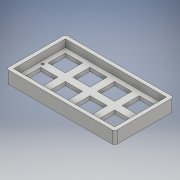
# Autodesk Inventor part: Key Plate
Saved by Autodesk Inventor 2018 (Build 220112000, 112)
## iProperties
Created: 2018-05-10
Part Number: Key Plate
Material: Generic
Document SubType Name: Modeling
Designer: mtsti
Density: 1 g/cm^3
Appearance: Default
Author: mtsti
Autodesk Inventor part; units mm, degrees
ref_plane "YZ Plane" through (0, 0, 0) normal (1, 0, 0) x (0, 1, 0)
ref_plane "XZ Plane" through (0, 0, 0) normal (0, 1, 0) x (-1, 0, 0)
ref_plane "XY Plane" through (0, 0, 0) normal (0, 0, 1) x (1, 0, 0)
sketch "Sketch1" plane through (0, 0, 0) normal (0, 0, 1) x (1, 0, 0)
  line L0 (3.0232, 17.5372) -> (17.0232, 17.5372)
  line L1 (17.0232, 17.5372) -> (17.0232, 3.5372)
  line L2 (17.0232, 3.5372) -> (3.0232, 3.5372)
  line L3 (3.0232, 3.5372) -> (3.0232, 17.5372)
  line L4 (3.0232, 23.5372) -> (17.0232, 23.5372)
  line L5 (17.0232, 23.5372) -> (17.0232, 37.5372)
  line L6 (17.0232, 37.5372) -> (3.0232, 37.5372)
  line L7 (3.0232, 37.5372) -> (3.0232, 23.5372)
  line L8 (23.0232, 17.5372) -> (37.0232, 17.5372)
  line L9 (37.0232, 17.5372) -> (37.0232, 3.5372)
  line L10 (37.0232, 3.5372) -> (23.0232, 3.5372)
  line L11 (23.0232, 3.5372) -> (23.0232, 17.5372)
  line L12 (23.0232, 23.5372) -> (37.0232, 23.5372)
  line L13 (37.0232, 23.5372) -> (37.0232, 37.5372)
  line L14 (37.0232, 37.5372) -> (23.0232, 37.5372)
  line L15 (23.0232, 37.5372) -> (23.0232, 23.5372)
  line L16 (43.0232, 17.5372) -> (57.0232, 17.5372)
  line L17 (57.0232, 17.5372) -> (57.0232, 3.5372)
  line L18 (57.0232, 3.5372) -> (43.0232, 3.5372)
  line L19 (43.0232, 3.5372) -> (43.0232, 17.5372)
  line L20 (43.0232, 23.5372) -> (57.0232, 23.5372)
  line L21 (57.0232, 23.5372) -> (57.0232, 37.5372)
  line L22 (57.0232, 37.5372) -> (43.0232, 37.5372)
  line L23 (43.0232, 37.5372) -> (43.0232, 23.5372)
  line L24 (63.0232, 17.5372) -> (77.0232, 17.5372)
  line L25 (77.0232, 17.5372) -> (77.0232, 3.5372)
  line L26 (77.0232, 3.5372) -> (63.0232, 3.5372)
  line L27 (63.0232, 3.5372) -> (63.0232, 17.5372)
  line L28 (63.0232, 23.5372) -> (77.0232, 23.5372)
  line L29 (77.0232, 23.5372) -> (77.0232, 37.5372)
  line L30 (77.0232, 37.5372) -> (63.0232, 37.5372)
  line L31 (63.0232, 37.5372) -> (63.0232, 23.5372)
  line L32 (1.0232, 1.5372) -> (79.0232, 1.5372)
  line L33 (79.0232, 1.5372) -> (79.0232, 39.5372)
  line L34 (79.0232, 39.5372) -> (1.0232, 39.5372)
  line L35 (1.0232, 39.5372) -> (1.0232, 1.5372)
  point P0 (0, 0)
  dimension "d0" = 14
  dimension "d1" = 14
  dimension "d2" = 14
  dimension "d3" = 14
  dimension "d4" = 6
  dimension "d5" = 14
  dimension "d6" = 14
  dimension "d7" = 14
  dimension "d8" = 14
  dimension "d9" = 6
  dimension "d10" = 6
  dimension "d11" = 0
  dimension "d12" = 14
  dimension "d13" = 14
  dimension "d14" = 14
  dimension "d15" = 14
  dimension "d16" = 6
  dimension "d17" = 14
  dimension "d18" = 14
  dimension "d19" = 14
  dimension "d20" = 14
  dimension "d21" = 6
  dimension "d22" = 6
  dimension "d23" = 0
  dimension "d24" = 6
  dimension "d25" = 0
  dimension "d26" = 2
  dimension "d27" = 2
  dimension "d28" = 2
  dimension "d29" = 2
  constraints: 72 end point, 18 parallel, 9 horizontal, 9 perpendicular, 4 point on line
  measures "d0" distance of L1.end L2.end
  measures "d1" distance of L0.end L1.end
  measures "d2" distance of L6.end L5.end
  measures "d3" distance of L5.end L4.end
  measures "d4" distance between parallel lines of L0 L4
  measures "d5" distance of L9.end L10.end
  measures "d6" distance of L8.end L9.end
  measures "d7" distance of L14.end L13.end
  measures "d8" distance of L13.end L12.end
  measures "d9" distance between parallel lines of L8 L12
  measures "d10" distance between parallel lines of L15 L5
  measures "d11" distance between parallel lines of L14 L6
  measures "d12" distance of L17.end L18.end
  measures "d13" distance of L16.end L17.end
  measures "d14" distance of L23.start L22.start
  measures "d15" distance of L22.start L20.end
  measures "d16" distance between parallel lines of L16 L20
  measures "d17" distance of L25.end L26.end
  measures "d18" distance of L24.end L25.end
  measures "d19" distance of L31.start L30.start
  measures "d20" distance of L30.start L28.end
  measures "d21" distance between parallel lines of L24 L28
  measures "d22" distance between parallel lines of L13 L23
  measures "d23" distance between parallel lines of L12 L20
  measures "d24" distance between parallel lines of L31 L21
  measures "d25" distance between parallel lines of L20 L28
  measures "d26" distance between parallel lines of L34 L6
  measures "d27" distance between parallel lines of L35 L7
  measures "d28" distance between parallel lines of L33 L25
  measures "d29" distance between parallel lines of L32 L26
sketch "Sketch3" plane through (0, 0, 0) normal (0, 0, 1) x (1, 0, 0)
  line L0 (3.0232, 17.5372) -> (17.0232, 17.5372)
  line L1 (17.0232, 17.5372) -> (17.0232, 3.5372)
  line L2 (17.0232, 3.5372) -> (3.0232, 3.5372)
  line L3 (3.0232, 3.5372) -> (3.0232, 17.5372)
  line L4 (3.0232, 23.5372) -> (17.0232, 23.5372)
  line L5 (17.0232, 23.5372) -> (17.0232, 37.5372)
  line L6 (17.0232, 37.5372) -> (3.0232, 37.5372)
  line L7 (3.0232, 37.5372) -> (3.0232, 23.5372)
  line L8 (23.0232, 17.5372) -> (37.0232, 17.5372)
  line L9 (37.0232, 17.5372) -> (37.0232, 3.5372)
  line L10 (37.0232, 3.5372) -> (23.0232, 3.5372)
  line L11 (23.0232, 3.5372) -> (23.0232, 17.5372)
  line L12 (23.0232, 23.5372) -> (37.0232, 23.5372)
  line L13 (37.0232, 23.5372) -> (37.0232, 37.5372)
  line L14 (37.0232, 37.5372) -> (23.0232, 37.5372)
  line L15 (23.0232, 37.5372) -> (23.0232, 23.5372)
  line L16 (43.0232, 17.5372) -> (57.0232, 17.5372)
  line L17 (57.0232, 17.5372) -> (57.0232, 3.5372)
  line L18 (57.0232, 3.5372) -> (43.0232, 3.5372)
  line L19 (43.0232, 3.5372) -> (43.0232, 17.5372)
  line L20 (43.0232, 23.5372) -> (57.0232, 23.5372)
  line L21 (43.0232, 37.5372) -> (43.0232, 23.5372)
  line L22 (57.0232, 37.5372) -> (43.0232, 37.5372)
  line L23 (57.0232, 23.5372) -> (57.0232, 37.5372)
  line L24 (63.0232, 17.5372) -> (77.0232, 17.5372)
  line L25 (77.0232, 17.5372) -> (77.0232, 3.5372)
  line L26 (77.0232, 3.5372) -> (63.0232, 3.5372)
  line L27 (63.0232, 3.5372) -> (63.0232, 17.5372)
  line L28 (63.0232, 23.5372) -> (77.0232, 23.5372)
  line L29 (63.0232, 37.5372) -> (63.0232, 23.5372)
  line L30 (77.0232, 37.5372) -> (63.0232, 37.5372)
  line L31 (77.0232, 23.5372) -> (77.0232, 37.5372)
  line L32 (1.0232, 1.5372) -> (79.0232, 1.5372)
  line L33 (79.0232, 1.5372) -> (79.0232, 39.5372)
  line L34 (79.0232, 39.5372) -> (1.0232, 39.5372)
  line L35 (1.0232, 39.5372) -> (1.0232, 1.5372)
  line L36 (-0.9768, -0.4628) -> (81.0232, -0.4628)
  line L37 (81.0232, -0.4628) -> (81.0232, 41.5372)
  line L38 (81.0232, 41.5372) -> (-0.9768, 41.5372)
  line L39 (-0.9768, 41.5372) -> (-0.9768, -0.4628)
  line L40 (-3.9768, 44.5372) -> (84.0232, 44.5372)
  line L41 (84.0232, 44.5372) -> (84.0232, -3.4628)
  line L42 (84.0232, -3.4628) -> (-3.9768, -3.4628)
  line L43 (-3.9768, -3.4628) -> (-3.9768, 44.5372)
  point P0 (0, 0)
  point P1 (0, 0)
  dimension "d31" = 14
  dimension "d32" = 14
  dimension "d33" = 14
  dimension "d34" = 14
  dimension "d35" = 6
  dimension "d36" = 14
  dimension "d37" = 14
  dimension "d38" = 14
  dimension "d39" = 14
  dimension "d40" = 6
  dimension "d41" = 6
  dimension "d42" = 0
  dimension "d43" = 14
  dimension "d44" = 14
  dimension "d45" = 14
  dimension "d46" = 14
  dimension "d47" = 6
  dimension "d48" = 14
  dimension "d49" = 14
  dimension "d50" = 14
  dimension "d51" = 14
  dimension "d52" = 6
  dimension "d53" = 6
  dimension "d54" = 0
  dimension "d55" = 6
  dimension "d56" = 0
  dimension "d57" = 2
  dimension "d58" = 2
  dimension "d59" = 2
  dimension "d60" = 2
  dimension "d61" = 2
  dimension "d62" = 2
  dimension "d63" = 2
  dimension "d64" = 2
  dimension "d65" = 3
  dimension "d66" = 3
  dimension "d67" = 3
  dimension "d68" = 3
  constraints: 88 end point, 22 parallel, 11 horizontal, 11 perpendicular, 4 point on line
  measures "d31" distance of L1.end L2.end
  measures "d32" distance of L0.end L1.end
  measures "d33" distance of L6.end L5.end
  measures "d34" distance of L5.end L4.end
  measures "d35" distance between parallel lines of L0 L4
  measures "d36" distance of L9.end L10.end
  measures "d37" distance of L8.end L9.end
  measures "d38" distance of L14.end L13.end
  measures "d39" distance of L13.end L12.end
  measures "d40" distance between parallel lines of L8 L12
  measures "d41" distance between parallel lines of L15 L5
  measures "d42" distance between parallel lines of L14 L6
  measures "d43" distance of L17.end L18.end
  measures "d44" distance of L16.end L17.end
  measures "d45" distance of L21.start L22.start
  measures "d46" distance of L22.start L20.end
  measures "d47" distance between parallel lines of L16 L20
  measures "d48" distance of L25.end L26.end
  measures "d49" distance of L24.end L25.end
  measures "d50" distance of L29.start L30.start
  measures "d51" distance of L30.start L28.end
  measures "d52" distance between parallel lines of L24 L28
  measures "d53" distance between parallel lines of L13 L21
  measures "d54" distance between parallel lines of L12 L20
  measures "d55" distance between parallel lines of L29 L23
  measures "d56" distance between parallel lines of L20 L28
  measures "d57" distance between parallel lines of L34 L6
  measures "d58" distance between parallel lines of L35 L7
  measures "d59" distance between parallel lines of L33 L25
  measures "d60" distance between parallel lines of L32 L26
  measures "d61" distance between parallel lines of L34 L38
  measures "d62" distance between parallel lines of L39 L35
  measures "d63" distance between parallel lines of L36 L32
  measures "d64" distance between parallel lines of L33 L37
  measures "d65" distance between parallel lines of L38 L40
  measures "d66" distance between parallel lines of L43 L39
  measures "d67" distance between parallel lines of L42 L36
  measures "d68" distance between parallel lines of L37 L41
extrude "Extrusion1" add sketch "Sketch3" against normal blind 3 contours L0 L1 L2 L3 | L7 L6 L5 L4 | L8 L9 L10 L11 | L15 L14 L13 L12 | L16 L17 L18 L19 | L21 L22 L23 L20 | L24 L25 L26 L27 | L29 L30 L31 L28 | L35 L34 L33 L32 | L39 L38 L37 L36 | L40 L41 L42 L43
extrude "Extrusion2" cut sketch "Sketch1" against normal blind 25 contours L0 L1 L2 L3 | L7 L6 L5 L4 | L8 L9 L10 L11 | L15 L14 L13 L12 | L16 L17 L18 L19 | L23 L22 L21 L20 | L24 L25 L26 L27 | L31 L30 L29 L28
sketch "Sketch4" plane through (0, 0, 0) normal (0, 0, 1) x (1, 0, 0)
  line L0 (-0.9768, 41.5372) -> (81.0232, 41.5372)
  line L1 (81.0232, 41.5372) -> (81.0232, -0.4628)
  line L2 (81.0232, -0.4628) -> (-0.9768, -0.4628)
  line L3 (-0.9768, -0.4628) -> (-0.9768, 41.5372)
  line L4 (84.0232, -3.4628) -> (-3.9768, -3.4628)
  line L5 (-3.9768, -3.4628) -> (-3.9768, 44.5372)
  line L6 (-3.9768, 44.5372) -> (84.0232, 44.5372)
  line L7 (84.0232, 44.5372) -> (84.0232, -3.4628)
  line L8 (23.0232, 37.5372) -> (37.0232, 37.5372) projected
  line L9 (3.0232, 23.5372) -> (3.0232, 37.5372) projected
  line L10 (17.0232, 3.5372) -> (3.0232, 3.5372) projected
  line L11 (77.0232, 37.5372) -> (77.0232, 23.5372) projected
  line L12 (-3.9768, 44.5372) -> (84.0232, 44.5372) projected
  line L13 (84.0232, 44.5372) -> (84.0232, -3.4628) projected
  line L14 (84.0232, -3.4628) -> (-3.9768, -3.4628) projected
  line L15 (-3.9768, -3.4628) -> (-3.9768, 44.5372) projected
  point P0 (0, 0)
  dimension "d73" = 4
  dimension "d74" = 4
  dimension "d75" = 4
  dimension "d76" = 4
  dimension "d77" = 0
  dimension "d78" = 0
  dimension "d79" = 0
  dimension "d80" = 0
  constraints: 16 end point, 4 parallel, 2 horizontal, 2 perpendicular
  measures "d73" distance between parallel lines of L8 L0
  measures "d74" distance between parallel lines of L9 L3
  measures "d75" distance between parallel lines of L2 L10
  measures "d76" distance between parallel lines of L1 L11
  measures "d77" distance between parallel lines of L12 L6
  measures "d78" distance between parallel lines of L7 L13
  measures "d79" distance between parallel lines of L14 L4
  measures "d80" distance between parallel lines of L15 L5
extrude "Extrusion3" add sketch "Sketch4" along normal blind 6
fillet "Fillet1" radius 2 4 edges at (-3.9768, 44.5372, 1.5) (84.0232, 44.5372, 1.5) (84.0232, -3.4628, 1.5) (-3.9768, -3.4628, 1.5)
sketch "Sketch5" plane through (0, 0, -3) normal (0, 0, -1) x (-1, 0, 0)
  line L0 (3.9768, -3.4628) -> (-84.0232, -3.4628)
  line L1 (-84.0232, -3.4628) -> (-84.0232, 44.5372)
  line L2 (-84.0232, 44.5372) -> (3.9768, 44.5372)
  line L3 (3.9768, 44.5372) -> (3.9768, -3.4628)
  line L4 (-82.0232, -3.4628) -> (1.9768, -3.4628) projected
  line L5 (-84.0232, 42.5372) -> (-84.0232, -1.4628) projected
  line L6 (1.9768, 44.5372) -> (-82.0232, 44.5372) projected
  line L7 (3.9768, -1.4628) -> (3.9768, 42.5372) projected
  line L8 (2.9768, -2.4628) -> (-83.0232, -2.4628)
  line L9 (-83.0232, -2.4628) -> (-83.0232, 43.5372)
  line L10 (-83.0232, 43.5372) -> (2.9768, 43.5372)
  line L11 (2.9768, 43.5372) -> (2.9768, -2.4628)
  point P0 (0, 0)
  dimension "d84" = 0
  dimension "d85" = 0
  dimension "d86" = 0
  dimension "d87" = 0
  dimension "d88" = 1
  dimension "d89" = 1
  dimension "d90" = 1
  dimension "d91" = 1
  constraints: 16 end point, 4 parallel, 2 horizontal, 2 perpendicular
  measures "d84" distance between parallel lines of L4 L0
  measures "d85" distance between parallel lines of L1 L5
  measures "d86" distance between parallel lines of L6 L2
  measures "d87" distance between parallel lines of L7 L3
  measures "d88" distance between parallel lines of L4 L8
  measures "d89" distance between parallel lines of L5 L9
  measures "d90" distance between parallel lines of L6 L10
  measures "d91" distance between parallel lines of L7 L11
extrude "Extrusion4" add sketch "Sketch5" along normal blind 1
fillet "Fillet2" radius 2 4 edges at (84.0232, -3.4628, -3.5) (84.0232, 44.5372, -3.5) (-3.9768, 44.5372, -3.5) (-3.9768, -3.4628, -3.5)
sketch "Sketch6" plane through (0, 0, 0) normal (0, 0, 1) x (1, 0, 0)
  circle A0 centre (1.5232, 20.5372) radius 1
  circle A1 centre (78.5232, 20.5372) radius 1
  line L0 (-0.9768, 41.5372) -> (81.0232, 41.5372) projected
  line L1 (-0.9768, -0.4628) -> (-0.9768, 41.5372) projected
  line L2 (77.0232, 23.5372) -> (63.0232, 23.5372) projected
  line L3 (81.0232, 41.5372) -> (81.0232, -0.4628) projected
  point P0 (0, 0)
  dimension "d95" = 2
  dimension "d96" = 2
  dimension "d97" = 21
  dimension "d98" = 2.5
  dimension "d99" = 3
  dimension "d100" = 2.5
  constraints: 2 centre point
  measures "d95" diameter of A0
  measures "d96" diameter of A1
  measures "d97" distance from line of L0 A0.centre
  measures "d98" distance from line of L1 A0.centre
  measures "d99" distance from line of A1.centre L2
  measures "d100" distance from line of L3 A1.centre
extrude "Extrusion5" cut sketch "Sketch6" against normal blind 10
body "Solid1"
